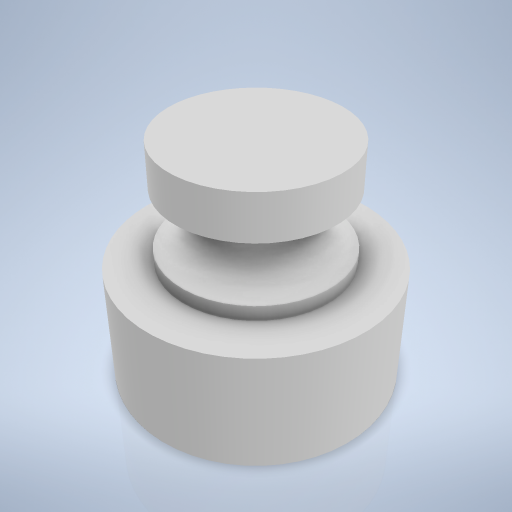
# Autodesk Inventor part: 7
Saved by Autodesk Inventor 2024.2 (Build 282272000, 272)
## iProperties
Created: 2024-05-04
Part Number: 7
Material: Generisch
Document SubType Name: Modeling
Designer: Fabri
Density: 1 g/cm^3
Appearance: Vorgabe
Author: Fabri
Autodesk Inventor part; units mm, degrees
ref_plane "XZ Plane" through (0, 0, 0) normal (0, 1, 0) x (-1, 0, 0)
ref_plane "XY Plane" through (0, 0, 0) normal (0, 0, 1) x (1, 0, 0)
sketch "Skizze1" plane through (0, 0, 0) normal (0, 0, 1) x (-1, 0, 0)
  circle A0 centre (0, 0) radius 22.5
  dimension "d0" = 45
  constraints: 1 centre point, 1 coincident
  measures "d0" diameter of A0
extrude "Extrusion1" add sketch "Skizze1" against normal blind 20
sketch "Skizze3" plane through (0, 0, 0) normal (0, 0, 1) x (1, 0, 0)
  circle A0 centre (0, 0) radius 15
  dimension "d3" = 30
  constraints: 1 centre point, 1 coincident
  measures "d3" diameter of A0
extrude "Extrusion2" add sketch "Skizze3" along normal blind 20
ref_plane "Arbeitsebene1" through (0, 0, 0) normal (1, 0, 0) x (0, 1, 0)
sketch "Skizze5" plane through (0, 0, 0) normal (1, 0, 0) x (0, 1, 0)
  line L0 (-22.5, -20) -> (22.5, -20) projected
  line L1 (0, -20) -> (0, 20)
  line L2 (15, 20) -> (-15, 20) projected
  line L3 (10, 20) -> (10, 1.8057) construction
  line L4 (10, 2.5) -> (10, 12.5)
  line L5 (15, 2.5) -> (15, 12.5)
  line L6 (15, 0) -> (15, 20) projected
  arc A0 (15, 12.5) -> (15, 2.5) centre (15, 7.5) ccw
  point P0 (0, 0)
  point P1 (10, 7.5)
  dimension "d8" = 20
  dimension "d10" = 7.5
  dimension "d13" = 5
  constraints: 8 end point, 4 point on line, 3 midpoint, 3 point on circle, 2 vertical, 1 centre point, 1 collinear, 1 horizontal alignment, 1 tangent
  measures "d8" diameter of L3 L1
  measures "d10" distance from line of L2 L4.end
  measures "d13" radius of A0
revolve "Umdrehung1" cut sketch "Skizze5" angle 360 about axis through (0, 0, -20) along (0, 0, 1)
